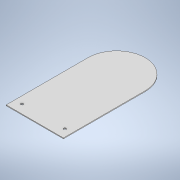
# Autodesk Inventor part: Magnetplatte
Saved by Autodesk Inventor 2022 (Build 260153000, 153)
## iProperties
Created: 2022-04-02
Part Number: Magnetplatte
Material: Generic
Document SubType Name: Modeling
Designer: benni
Density: 1 g/cm^3
Appearance: Default
Author: benni
Autodesk Inventor part; units mm, degrees
ref_plane "YZ Plane" through (0, 0, 0) normal (1, 0, 0) x (0, 1, 0)
ref_plane "XZ Plane" through (0, 0, 0) normal (0, 1, 0) x (-1, 0, 0)
ref_plane "XY Plane" through (0, 0, 0) normal (0, 0, 1) x (1, 0, 0)
sketch "Sketch1" plane through (0, 0, 0) normal (0, 1, 0) x (-1, 0, 0)
  line L0 (33.1684, 49.7042) -> (-36.8316, 49.7042)
  line L1 (-36.8316, 49.7042) -> (-36.8316, -50.2958)
  line L2 (-36.8316, -50.2958) -> (33.1684, -50.2958)
  line L3 (33.1684, -50.2958) -> (33.1684, 49.7042)
  arc A0 (-36.8316, -50.2958) -> (33.1684, -50.2958) centre (-1.8316, -50.2958) ccw
  circle A1 centre (24.4184, 39.2042) radius 1.5
  circle A2 centre (-28.0816, 39.2042) radius 1.5
  point P0 (0, 0)
  dimension "d0" = 100
  dimension "d1" = 70
  dimension "d2" = 10.5
  dimension "d4" = 10.5
  dimension "d8" = 3
  dimension "d9" = 3
  dimension "d12" = 52.5
  constraints: 8 end point, 4 coincident, 3 centre point, 2 parallel, 2 point on circle, 1 horizontal, 1 midpoint, 1 perpendicular, 1 point on line
  measures "d0" distance of L3.end L2.end
  measures "d1" distance of L1.end L2.end
  measures "d2" distance from line of L0 point (24.418, 39.204)
  measures "d4" distance from line of L0 point (-28.082, 39.204)
  measures "d8" diameter of A1
  measures "d9" diameter of A2
  measures "d12" distance of A2.centre point (24.418, 39.204)
extrude "Extrusion1" add sketch "Sketch1" along normal blind 1
body "Solid1"
